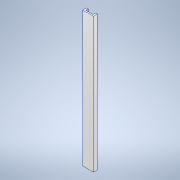
# Autodesk Inventor part: L_PlNKA800
Saved by Autodesk Inventor 2022 (Build 260153000, 153)
## iProperties
Created: 2023-08-15
Part Number: L_PlNKA800
Material: Aluminum 6061
Document SubType Name: Modeling
Designer: Kippi
Mass: 3520.8 g
Surface Area: 2546.08 cm^2
Volume: 1304 cm^3
Density: 2.7 g/cm^3
Appearance: Aluminum - Flat
Author: Kippi
Autodesk Inventor part; units mm, degrees
ref_plane "YZ Plane" through (0, 0, 0) normal (1, 0, 0) x (0, 1, 0)
ref_plane "XZ Plane" through (0, 0, 0) normal (0, 1, 0) x (-1, 0, 0)
ref_plane "XY Plane" through (0, 0, 0) normal (0, 0, 1) x (1, 0, 0)
sketch "Sketch1" plane through (0, 0, 0) normal (0, 1, 0) x (-1, 0, 0)
  line L0 (10, 6) -> (-70, 6)
  line L1 (-70, 6) -> (-70, -9)
  line L2 (-70, -9) -> (10, -9)
  line L3 (10, -9) -> (10, 6)
  line L4 (-17, -9) -> (-4, -22)
  line L5 (-4, -22) -> (10, -22)
  line L6 (10, -22) -> (10, -9)
  line L7 (-43, -9) -> (-56, -22)
  line L8 (-56, -22) -> (-70, -22)
  line L9 (-70, -22) -> (-70, -9)
  line L10 (-56, -22) -> (-4, -22)
  line L11 (-4, -22) -> (-4, -4)
  line L12 (-4, -4) -> (-56, -4)
  line L13 (-56, -4) -> (-56, -22)
  point P0 (0, 0)
  point P1 (-4, -22)
  dimension "d0" = 15
  dimension "d1" = 80
  constraints: 28 end point, 5 perpendicular, 4 parallel, 4 point on line, 3 horizontal
  measures "d0" distance of L2.end L0.start
  measures "d1" distance of L1.end L2.end
extrude "Extrusion1" add sketch "Sketch1" along normal blind 1000 contours L3 L2 L11 L12 L13 L1 L0 | L6 L5 L11 L2 | L2 L13 L8 L9
body "Solid1"
